Autodesk Fusion 360 part; units mm, degrees
(part 2 of 2)
  line L12 (-35.657, -37.3371) -> (-35.6719, -36.3198)
  spline S215 degree 2 poles (-35.6719, -36.3198) (-33.6544, -34.0879) (-32.0207, -32.0895) knots 0 0 0 1 1 1
  spline S216 degree 2 poles (-32.0207, -32.0895) (-30.387, -30.0911) (-29.5009, -28.8935) knots 0 0 0 1 1 1
  spline S217 degree 2 poles (-29.5009, -28.8935) (-28.6148, -27.6958) (-28.4659, -27.4962) knots 0 0 0 1 1 1
  spline S218 degree 2 poles (-28.4659, -27.4962) (-28.0637, -26.9587) (-27.744, -26.4908) knots 0 0 0 1 1 1
  spline S219 degree 2 poles (-27.744, -26.4908) (-27.4244, -26.0229) (-27.2079, -25.7691) knots 0 0 0 1 1 1
  spline S220 degree 2 poles (-27.2079, -25.7691) (-26.9914, -25.5153) (-26.8547, -25.5133) knots 0 0 0 1 1 1
  spline S221 degree 2 poles (-26.8547, -25.5133) (-26.5359, -25.5086) (-26.2761, -26.1351) knots 0 0 0 1 1 1
  spline S222 degree 2 poles (-26.2761, -26.1351) (-26.0163, -26.7616) (-26.0091, -27.2475) knots 0 0 0 1 1 1
  spline S223 degree 2 poles (-26.0091, -27.2475) (-26.0027, -27.6878) (-26.1648, -28.0244) knots 0 0 0 1 1 1
  spline S224 degree 2 poles (-26.1648, -28.0244) (-27.2219, -30.5003) (-30.9438, -36.6452) knots 0 0 0 1 1 1
emboss "Emboss1" depth 5 profiles "Sketch5" section 1 onto face at (49.7515, 147.0216, 66.6667) on bodies 2 bodies 2
sketch "Sketch6" plane through (0, 0, 100) normal (0, 0, 1) x (-1, 0, 0)
  circle A0 centre (0, -152) radius 50
sketch "Sketch7" plane through (0, 0, 100) normal (0, 0, 1) x (-1, 0, 0)
  circle A0 centre (0, -152) radius 50
  circle A1 centre (0, -152) radius 48
  dimension "d26" = -2
extrude "Extrude2" cut sketch "Sketch7" against normal through all contours A1 bodies 2
